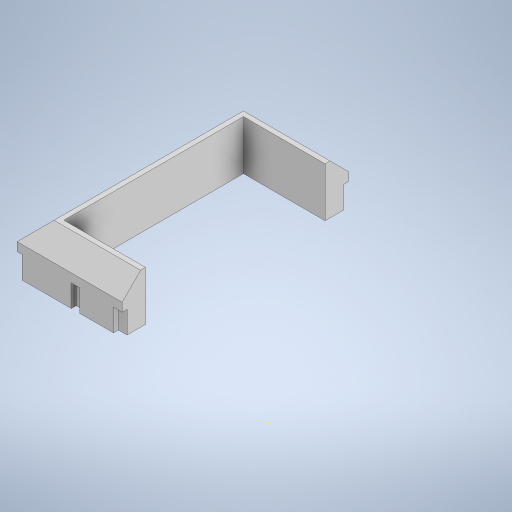
# Autodesk Inventor part: Palm_FingerAttachment
Saved by Autodesk Inventor 2023 (Build 270158000, 158)
## iProperties
Created: 2023-04-19
Part Number: Palm_FingerAttachment
Material: Generic
Document SubType Name: Modeling
Designer: 1senadi
Density: 1 g/cm^3
Appearance: Default
Author: 1senadi
Autodesk Inventor part; units mm, degrees
ref_plane "YZ Plane" through (0, 0, 0) normal (1, 0, 0) x (0, 1, 0)
ref_plane "XZ Plane" through (0, 0, 0) normal (0, 1, 0) x (-1, 0, 0)
ref_plane "XY Plane" through (0, 0, 0) normal (0, 0, 1) x (1, 0, 0)
sketch "Sketch1" plane through (0, 0, 0) normal (0, 1, 0) x (-1, 0, 0)
  line L0 (0, 0) -> (102, 0)
  line L1 (102, 0) -> (102, 91.8)
  line L2 (102, 91.8) -> (0, 91.8)
  line L3 (0, 91.8) -> (0, 0)
  line L4 (92.5, 82.3) -> (92.5, 9.5)
  line L5 (92.5, 9.5) -> (9.5, 9.5)
  line L6 (9.5, 9.5) -> (9.5, 82.3)
  line L7 (9.5, 82.3) -> (92.5, 82.3)
  dimension "d0" = 102
  dimension "d1" = 91.8
  dimension "d2" = 9.5
  constraints: 16 end point, 4 parallel, 2 perpendicular, 1 horizontal, 3 other
  measures "d0" distance of L2.end L1.end
  measures "d1" distance of L1.end L0.end
  measures "d2" distance between parallel lines of L1 L4
extrude "Extrusion1" add sketch "Sketch1" along normal blind 20
sketch "Sketch2" plane through (-102, 0, 0) normal (-1, 0, 0) x (0, 0, 1)
  line L0 (0, 0) -> (0, 9)
  line L1 (0, 0) -> (0, 20) projected
  line L2 (0, 9) -> (3.5, 9)
  line L3 (3.5, 9) -> (3.5, 0)
  line L4 (91.8, 0) -> (0, 0) projected
  line L5 (0, 0) -> (3.5, 0)
  line L6 (3.5, 0) -> (17.1, 0)
  line L7 (17.1, 0) -> (17.1, 9)
  line L8 (17.1, 9) -> (20.6, 9)
  line L9 (20.6, 9) -> (20.6, 0)
  line L10 (17.1, 0) -> (20.6, 0)
  line L11 (56.2, 9) -> (56.2, 0)
  line L12 (52.7, 9) -> (56.2, 9)
  line L13 (52.7, 0) -> (52.7, 9)
  line L14 (52.7, 0) -> (56.2, 0)
  line L15 (39.1, 0) -> (52.7, 0)
  line L16 (39.1, 9) -> (39.1, 0)
  line L17 (35.6, 9) -> (39.1, 9)
  line L18 (35.6, 0) -> (35.6, 9)
  line L19 (35.6, 0) -> (39.1, 0)
  line L20 (91.8, 9) -> (91.8, 0)
  line L21 (88.3, 9) -> (91.8, 9)
  line L22 (88.3, 0) -> (88.3, 9)
  line L23 (88.3, 0) -> (91.8, 0)
  line L24 (74.7, 0) -> (88.3, 0)
  line L25 (74.7, 9) -> (74.7, 0)
  line L26 (71.2, 9) -> (74.7, 9)
  line L27 (71.2, 0) -> (71.2, 9)
  line L28 (71.2, 0) -> (74.7, 0)
  point P0 (88.3, 0)
  point P1 (74.7, 0)
  point P2 (52.7, 0)
  point P3 (39.1, 0)
  dimension "d5" = 9
  dimension "d6" = 3.5
  dimension "d7" = 13.6
  dimension "d8" = 9
  dimension "d9" = 3.5
  dimension "d12" = 35.6
  constraints: 54 end point, 6 perpendicular, 4 point on line, 1 collinear, 1 horizontal, 34 other
  measures "d5" distance of L0.start L0.end
  measures "d6" distance of L0.end L2.end
  measures "d7" distance of L3.end L6.end
  measures "d8" distance of L6.end L7.end
  measures "d9" distance of L7.end L8.end
  measures "d12" distance of L8.end L11.start
extrude "Extrusion2" cut sketch "Sketch2" against normal blind 2
sketch "Sketch3" plane through (-102, 20, 91.8) normal (0, 0, 1) x (1, 0, 0)
  point P0 (102, -20)
sketch "Sketch4" plane through (-102, 20, 91.8) normal (0, 0, 1) x (1, 0, 0)
  line L0 (2, -20) -> (0, -20) projected
  line L1 (2, -20) -> (22, -20)
  line L2 (9.5, -20) -> (92.5, -20) projected
  line L3 (22, -20) -> (22, -11)
  line L4 (22, -11) -> (25.5, -11)
  line L5 (25.5, -11) -> (25.5, -20)
  line L6 (22, -20) -> (25.5, -20)
  line L7 (25.5, -20) -> (39.1, -20)
  line L8 (39.1, -20) -> (39.1, -11)
  line L9 (39.1, -11) -> (42.6, -11)
  line L10 (42.6, -11) -> (42.6, -20)
  line L11 (42.6, -20) -> (39.1, -20)
  point P0 (102, -20)
  dimension "d19" = 20
  dimension "d20" = 9
  dimension "d21" = 3.5
  dimension "d22" = 13.6
  dimension "d23" = 9
  dimension "d24" = 3.5
  constraints: 20 end point, 6 point on line, 3 perpendicular, 2 collinear, 1 vertical
  measures "d19" distance of L0.start L1.end
  measures "d20" distance of L1.end L3.end
  measures "d21" distance of L3.end L4.end
  measures "d22" distance of L5.end L7.end
  measures "d23" distance of L7.end L8.end
  measures "d24" distance of L8.end L9.end
extrude "Extrusion3" cut sketch "Sketch4" against normal blind 2
ref_plane "Work Plane1" through (-102, 0, 45.9) normal (0, 0, 1) x (1, 0, 0)
mirror "Mirror1" about plane through (-102, 0, 45.9) normal (0, 0, 1) of "Extrusion3"
sketch "Sketch5" plane through (0, 0, 0) normal (0, -1, 0) x (1, 0, 0)
  line L0 (-59.4, 2) -> (-59.4, 0) projected
  line L1 (0, 0) -> (-59.4, 0) projected
  line L2 (0, 91.8) -> (0, 0) projected
  line L3 (-59.4, 91.8) -> (0, 91.8) projected
  line L4 (-59.4, 91.8) -> (-59.4, 89.8) projected
  line L5 (-59.4, 89.8) -> (-62.9, 89.8) projected
  line L6 (-62.9, 89.8) -> (-62.9, 91.8) projected
  line L7 (-76.5, 91.8) -> (-62.9, 91.8) projected
  line L8 (-76.5, 91.8) -> (-76.5, 89.8) projected
  line L9 (-76.5, 89.8) -> (-80, 89.8) projected
  line L10 (-80, 89.8) -> (-80, 91.8) projected
  line L11 (-100, 91.8) -> (-80, 91.8) projected
  line L12 (-100, 91.8) -> (-100, 88.3) projected
  line L13 (-100, 88.3) -> (-102, 88.3) projected
  line L14 (-102, 74.7) -> (-102, 88.3) projected
  line L15 (-102, 74.7) -> (-100, 74.7) projected
  line L16 (-100, 74.7) -> (-100, 71.2) projected
  line L17 (-100, 71.2) -> (-102, 71.2) projected
  line L18 (-102, 56.2) -> (-102, 71.2) projected
  line L19 (-102, 56.2) -> (-100, 56.2) projected
  line L20 (-100, 56.2) -> (-100, 52.7) projected
  line L21 (-100, 52.7) -> (-102, 52.7) projected
  line L22 (-102, 39.1) -> (-102, 52.7) projected
  line L23 (-102, 39.1) -> (-100, 39.1) projected
  line L24 (-100, 39.1) -> (-100, 35.6) projected
  line L25 (-100, 35.6) -> (-102, 35.6) projected
  line L26 (-102, 20.6) -> (-102, 35.6) projected
  line L27 (-102, 20.6) -> (-100, 20.6) projected
  line L28 (-100, 20.6) -> (-100, 17.1) projected
  line L29 (-100, 17.1) -> (-102, 17.1) projected
  line L30 (-102, 3.5) -> (-102, 17.1) projected
  line L31 (-102, 3.5) -> (-100, 3.5) projected
  line L32 (-100, 3.5) -> (-100, 0) projected
  line L33 (-80, 0) -> (-100, 0) projected
  line L34 (-80, 0) -> (-80, 2) projected
  line L35 (-80, 2) -> (-76.5, 2) projected
  line L36 (-76.5, 2) -> (-76.5, 0) projected
  line L37 (-62.9, 0) -> (-76.5, 0) projected
  line L38 (-62.9, 0) -> (-62.9, 2) projected
  line L39 (-62.9, 2) -> (-59.4, 2) projected
  line L40 (-92.5, 82.3) -> (-92.5, 9.5) projected
  line L41 (-9.5, 82.3) -> (-92.5, 82.3) projected
  line L42 (-9.5, 9.5) -> (-9.5, 82.3) projected
  line L43 (-92.5, 9.5) -> (-9.5, 9.5) projected
  line L44 (-59.4, 0) -> (-59.4, 2) projected
  line L45 (-59.4, 91.8) -> (-59.4, 89.8) projected
  line L46 (-59.4, 0) -> (-59.4, 91.8)
  line L47 (-102, 91.8) -> (0, 91.8) projected
  line L48 (-59.4, 91.8) -> (0, 91.8)
  line L49 (0, 91.8) -> (0, 0)
  line L50 (0, 0) -> (-102, 0) projected
  line L51 (-59.4, 0) -> (0, 0)
  constraints: 8 end point, 1 collinear, 1 perpendicular
extrude "Extrusion4" cut sketch "Sketch5" against normal up to surface (20 mm away) contours L46 L43 L42 L41 L4 L3 L2 L1 L0 | L46 L41 L42 L43
sketch "Sketch6" plane through (-102, 9, 91.8) normal (0, 0, 1) x (1, 0, 0)
  line L0 (0, 11) -> (42.6, 11) projected
  line L1 (0, 11) -> (0, 3.5)
  line L2 (0, 0) -> (0, 11) projected
  line L3 (0, 3.5) -> (7.5, 11)
  line L4 (7.5, 11) -> (0, 11)
  point P0 (102, -9)
  point P1 (7.5, 11)
  dimension "d29" = 7.5
  dimension "d30" = 45
  constraints: 6 end point, 1 perpendicular, 1 point on line
  measures "d29" distance of L0.start L1.end
  measures "d30" angle of L3 L1
extrude "Extrusion5" cut sketch "Sketch6" against normal up to surface (91.8 mm away)
sketch "Sketch7" plane through (-59.4, 0, 89.8) normal (1, 0, 0) x (0, 0, -1)
  line L0 (-2, 20) -> (7.5, 20) projected
  line L1 (-2, 20) -> (-2, 12.5)
  line L2 (-2, 9) -> (-2, 20) projected
  line L3 (-2, 20) -> (5.5, 20) construction
  line L4 (-2, 12.5) -> (5.5, 20)
  line L5 (5.5, 20) -> (-2, 20)
  line L6 (7.5, 20) -> (80.3, 20) projected
  line L7 (43.9, 20) -> (43.9, -0.4844)
  line L8 (89.8, 20) -> (80.3, 20)
  line L9 (89.8, 20) -> (89.8, 12.5)
  line L10 (89.8, 12.5) -> (82.3, 20)
  point P0 (89.8, 0)
  dimension "d33" = 7.5
  dimension "d34" = 90
  dimension "d35" = 45
  constraints: 16 end point, 3 symmetric about line, 2 perpendicular, 1 collinear, 1 horizontal, 1 midpoint, 1 vertical
  measures "d33" distance of L0.start L1.end
  measures "d34" angle of L1 L3
  measures "d35" angle of L4 L1
extrude "Extrusion6" cut sketch "Sketch7" against normal up to surface (42.6 mm away)
body "Solid1"
